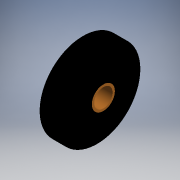
# Autodesk Inventor part: 25-2281_w
Saved by Autodesk Inventor 2017.3 (Build 213256000, 256)
## iProperties
Part Number: 25-2281_w
Material: Generic
Catalog Web Link: www.cadenas.de
Description: 25-2281, 65-2282, 40-2280, 40-2290_w-Roller Wheels
Vendor: 8020
Document SubType Name: Modeling
Designer: partserver
Manufacturer: 8020
Mass: 9.54074 g
Surface Area: 35.97 cm^2
Volume: 9.54074 cm^3
Density: 1 g/cm^3
Appearance: PSOLRGB-192-192-192
Category: PARTsolutions
Company: 8020
Title: 25-2281_w
Author: Cadenas PARTsolutions
Comments: Roller Wheels
PSOL_IDENT_0: {$CADENAS_DATA\23d-libs\8020\metric\linear_motion\25_2281.prj},193 {VTYP=3D},{NB=25-2281_w},{LINA=25
PSOL_IDENT_1: -2281_w},{NN=25-2281, 65-2282, 40-2280, 40-2290_w},{DATE=31.07.2020 09:21:29},{GEOMDATE=01.08.2013 1
PSOL_IDENT_2: 2:16:00},{VERSION=},{LINEID=10},{WBVAR=BT,RI},{WBNUMERIC=}  {NB=25-2281_w},{LINA=25-2281_w},{KT=DUMM
PSOL_IDENT_3: Y},{PN=25-2281},{NO=1},{MAT=Self-lubricating, fiberglass-reinforced black nylon.},{BT=2},{BT1= '2','
PSOL_IDENT_4: Permanent Lubricated Bronze Bushing' },{MT=25 Series},{RI=25},{RI1= '25','25 Series','40','40 Series'
PSOL_IDENT_5: },{A=37.500},{B=28.000},{C=6.100},{D=11.600},{E=14.000},{F=4.750},{G=8.000},{H=5.500},{J=3.200},{K=
PSOL_IDENT_6: 15.900},{L=13.200},{M=6.800},{N=M6 x 1.0},{N1=6.0000},{P=1.600},{Q=9.200},{W=.032},{G1=10.000},{K1=0
PSOL_IDENT_7: .000},{NTP=25-3382}
NB: 25-2281_w
NN: 25-2281, 65-2282, 40-2280, 40-2290_w
NT: Roller Wheels
NBSYN: $PN._w
LINA: 25-2281_w
CATALOG: 80/20
NO: 1
MAT: Self-lubricating, fiberglass-reinforced black nylon.
BT: Permanent Lubricated Bronze Bushing
MT: 25 Series
RI: 25 Series
A: 37.5
B: 28
D: 11.6
E: 14
F: 4.75
G: 8
H: 5.5
J: 3.2
K: 15.9
L: 13.2
M: 6.8
N: M6 x 1.0
N1: 6
P: 1.6
Q: 9.2
K1: 0
NTP: 25-3382
SUPPLIER: 8020
ARTICLENO: 25-2281_w
BOMINFO: 25-2281_w
CREATOR: CADENAS GmbH
Autodesk Inventor part; units mm, degrees
sketch "Sketch_1" plane through (0, 0, 0) normal (0, 0, 1) x (1, 0, 0)
  line L0 (5.8, 0) -> (-5.8, 0)
  line L1 (-5.8, 5.02) -> (-5.78, 5)
  line L2 (-5.78, 5) -> (5.78, 5)
  line L3 (5.78, 5) -> (5.8, 5.02)
  line L4 (5.8, 5.02) -> (5.8, 13.98)
  line L5 (5.8, 13.98) -> (5.78, 14)
  line L6 (5.78, 14) -> (3.081, 14)
  arc A0 (3.05, 14.031) -> (3.081, 14) centre (3.081, 14.031) ccw
  line L7 (3.05, 14.031) -> (3.05, 18.73)
  line L8 (3.05, 18.73) -> (3.03, 18.75)
  line L9 (3.03, 18.75) -> (-3.03, 18.75)
  line L10 (-3.03, 18.75) -> (-3.05, 18.73)
  line L11 (-3.05, 18.73) -> (-3.05, 14.031)
  arc A1 (-3.081, 14) -> (-3.05, 14.031) centre (-3.081, 14.031) ccw
  line L12 (-3.081, 14) -> (-5.78, 14)
  line L13 (-5.78, 14) -> (-5.8, 13.98)
  line L14 (-5.8, 13.98) -> (-5.8, 5.02)
  constraints: 30 end point, 4 point on circle, 2 centre point
revolve "Revolution1" add sketch "Sketch_1" angle 360 about axis through (5.8, 0, 0) along (1, 0, 0)
sketch "Sketch_2" plane through (0, 0, 0) normal (0, 0, 1) x (1, 0, 0)
  line L0 (5.8, 0) -> (-5.8, 0)
  line L1 (-5.8, 5) -> (-5.8, 4)
  line L2 (-5.8, 4) -> (5.8, 4)
  line L3 (5.8, 4) -> (5.8, 5)
  line L4 (5.8, 5) -> (-5.8, 5)
  constraints: 10 end point
revolve "Revolution2" add sketch "Sketch_2" angle 360 about axis through (5.8, 0, 0) along (1, 0, 0)
ref_plane "to_bolt_XY" through (5.8, 0, 0) normal (1, 0, 0) x (0, 0, -1)
ref_plane "to_bolt_YZ" through (5.8, 0, 0) normal (0, 0, -1) x (0, 1, 0)
ref_plane "to_bolt_ZX" through (5.8, 0, 0) normal (0, 1, 0) x (1, 0, 0)
ref_plane "wheel_XY" through (0, 0, 0) normal (1, 0, 0) x (0, 0, -1)
ref_plane "wheel_YZ" through (0, 0, 0) normal (0, 0, -1) x (0, 1, 0)
ref_plane "wheel_ZX" through (0, 0, 0) normal (0, 1, 0) x (1, 0, 0)
body "Solid1"
